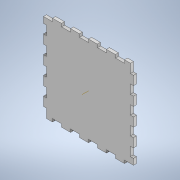
# Autodesk Inventor part: Lukt_hlidarplata
Saved by Autodesk Inventor 2021 (Build 250183000, 183)
## iProperties
Created: 2023-02-22
Part Number: Lukt_hlidarplata
Material: Generic
Document SubType Name: Modeling
Designer: frost
Density: 1 g/cm^3
Appearance: Default
width: 120.000 mm
height: 120.000 mm
thickness: 4.000 mm
finger: 12.000 mm
kerf: 0.220 mm
nr_width: 10.000 ul
nr_height: 10.000 ul
Author: frost
Autodesk Inventor part; units mm, degrees
ref_plane "YZ Plane" through (0, 0, 0) normal (1, 0, 0) x (0, 1, 0)
ref_plane "XZ Plane" through (0, 0, 0) normal (0, 1, 0) x (-1, 0, 0)
ref_plane "XY Plane" through (0, 0, 0) normal (0, 0, 1) x (1, 0, 0)
sketch "Sketch1" plane through (0, 0, 0) normal (0, 0, 1) x (1, 0, 0)
  line L0 (-60, -60) -> (60, -60)
  line L1 (60, -60) -> (60, 60)
  line L2 (60, 60) -> (-60, 60)
  line L3 (-60, 60) -> (-60, -60)
  line L4 (-30, 60) -> (-24.8931, 60)
  point P0 (0, 0)
  dimension "d0" = 120
  dimension "d1" = 120
  dimension "d2" = 60
  dimension "d3" = 60
  constraints: 10 end point, 2 horizontal, 2 parallel, 1 perpendicular, 1 point on line
  measures "d0" distance of L1.end L2.end
  measures "d1" distance of L0.end L1.end
  measures "d2" distance from line of L3 point (0, 0)
  measures "d3" distance from line of L2 point (0, 0)
extrude "Extrusion1" add sketch "Sketch1" along normal mid plane 4
sketch "Sketch3" plane through (-60, 60, 2) normal (0, 1, 0) x (1, 0, 0)
  line L0 (120, 0) -> (0, 0) projected
  line L1 (0, 4) -> (120, 4) projected
  line L2 (0, 0) -> (12, 0)
  line L3 (12, 0) -> (12, 4)
  line L4 (12, 4) -> (0, 4)
  line L5 (0, 4) -> (0, 0)
  line L6 (0, 4) -> (0, 0) projected
  point P0 (60, 2)
  dimension "d17" = 0
  dimension "d18" = 12
  constraints: 8 end point, 2 parallel, 2 point on line, 1 horizontal, 1 perpendicular
  measures "d17" distance between parallel lines of L6 L5
  measures "d18" distance between parallel lines of L3 L5
extrude "Extrusion2" cut sketch "Sketch3" against normal blind 4
pattern_linear "side_top" count 5 spacing 24 along (1, 0, 0) of "Extrusion2"
sketch "Sketch4" plane through (-60, 56, -2) normal (-1, 0, 0) x (0, 0, 1)
  line L0 (4, 0) -> (4, -116) projected
  line L1 (0, -116) -> (4, -116)
  line L2 (4, -116) -> (4, -104)
  line L3 (4, -104) -> (0, -104)
  line L4 (0, -104) -> (0, -116)
  line L5 (0, -116) -> (4, -116) projected
  point P0 (2, -56)
  point P1 (4, -112)
  point P2 (4, -104)
  dimension "d49" = 4
  dimension "d50" = 12
  dimension "d51" = 0
  dimension "d52" = 0
  constraints: 8 end point, 2 parallel, 1 horizontal, 1 perpendicular
  measures "d49" distance of L2.end L3.end
  measures "d50" distance of L3.end L1.start
  measures "d51" distance between parallel lines of L0 L2
  measures "d52" distance between parallel lines of L5 L1
extrude "Extrusion3" cut sketch "Sketch4" against normal blind 4
pattern_circular "side_bottom" count 2 over 360 about axis through (0, 0, -10) along (0, 0, 1) of "Extrusion2", "side_top"
pattern_linear "side_left" count 5 spacing 24 along (0, 1, 0) of "Extrusion3"
pattern_circular "side_right" count 2 over 360 about axis through (0, 0, -10) along (0, 0, 1) of "Extrusion3", "side_left"
sketch "Sketch6" plane through (0, 0, 2) normal (0, 0, 1) x (1, 0, 0)
  line L0 (60, -12) -> (60, 0) projected
  line L1 (60, 0) -> (56, 0) projected
  line L2 (56, 0) -> (56, 12) projected
  line L3 (56, 12) -> (60, 12) projected
  line L4 (60, 12) -> (60, 24) projected
  line L5 (60, 24) -> (56, 24) projected
  line L6 (56, 24) -> (56, 36) projected
  line L7 (56, 36) -> (60, 36) projected
  line L8 (60, 36) -> (60, 48) projected
  line L9 (60, 48) -> (56, 48) projected
  line L10 (56, 48) -> (56, 60) projected
  line L11 (56, 60) -> (48, 60) projected
  line L12 (48, 60) -> (48, 56) projected
  line L13 (48, 56) -> (36, 56) projected
  line L14 (36, 56) -> (36, 60) projected
  line L15 (36, 60) -> (24, 60) projected
  line L16 (24, 60) -> (24, 56) projected
  line L17 (24, 56) -> (12, 56) projected
  line L18 (12, 56) -> (12, 60) projected
  line L19 (12, 60) -> (0, 60) projected
  line L20 (0, 60) -> (0, 56) projected
  line L21 (0, 56) -> (-12, 56) projected
  line L22 (-12, 56) -> (-12, 60) projected
  line L23 (-12, 60) -> (-24, 60) projected
  line L24 (-24, 60) -> (-24, 56) projected
  line L25 (-24, 56) -> (-36, 56) projected
  line L26 (-36, 56) -> (-36, 60) projected
  line L27 (-36, 60) -> (-48, 60) projected
  line L28 (-48, 60) -> (-48, 56) projected
  line L29 (-48, 56) -> (-60, 56) projected
  line L30 (-60, 12) -> (-60, 0) projected
  line L31 (-60, 0) -> (-56, 0) projected
  line L32 (-56, 0) -> (-56, -12) projected
  line L33 (-56, -12) -> (-60, -12) projected
  line L34 (-60, -12) -> (-60, -24) projected
  line L35 (-60, -24) -> (-56, -24) projected
  line L36 (-56, -24) -> (-56, -36) projected
  line L37 (-56, -36) -> (-60, -36) projected
  line L38 (-60, -36) -> (-60, -48) projected
  line L39 (-60, -48) -> (-56, -48) projected
  line L40 (-56, -48) -> (-56, -60) projected
  line L41 (-56, -60) -> (-48, -60) projected
  line L42 (-48, -60) -> (-48, -56) projected
  line L43 (-48, -56) -> (-36, -56) projected
  line L44 (-36, -56) -> (-36, -60) projected
  line L45 (-36, -60) -> (-24, -60) projected
  line L46 (-24, -60) -> (-24, -56) projected
  line L47 (-24, -56) -> (-12, -56) projected
  line L48 (-12, -56) -> (-12, -60) projected
  line L49 (-12, -60) -> (0, -60) projected
  line L50 (0, -60) -> (0, -56) projected
  line L51 (0, -56) -> (12, -56) projected
  line L52 (12, -56) -> (12, -60) projected
  line L53 (12, -60) -> (24, -60) projected
  line L54 (24, -60) -> (24, -56) projected
  line L55 (24, -56) -> (36, -56) projected
  line L56 (36, -56) -> (36, -60) projected
  line L57 (36, -60) -> (48, -60) projected
  line L58 (48, -60) -> (48, -56) projected
  line L59 (48, -56) -> (60, -56) projected
  line L60 (-60.11, 60.11) -> (-35.89, 60.11)
  line L61 (-35.89, 60.11) -> (-35.89, 56.11)
  line L62 (-35.89, 56.11) -> (-24.11, 56.11)
  line L63 (-24.11, 56.11) -> (-24.11, 60.11)
  line L64 (-24.11, 60.11) -> (-11.89, 60.11)
  line L65 (-11.89, 60.11) -> (-11.89, 56.11)
  line L66 (-11.89, 56.11) -> (-0.11, 56.11)
  line L67 (-0.11, 56.11) -> (-0.11, 60.11)
  line L68 (-0.11, 60.11) -> (12.11, 60.11)
  line L69 (12.11, 60.11) -> (12.11, 56.11)
  line L70 (12.11, 56.11) -> (23.89, 56.11)
  line L71 (23.89, 56.11) -> (23.89, 60.11)
  line L72 (23.89, 60.11) -> (36.11, 60.11)
  line L73 (36.11, 60.11) -> (36.11, 56.11)
  line L74 (36.11, 56.11) -> (47.89, 56.11)
  line L75 (47.89, 56.11) -> (47.89, 60.11)
  line L76 (47.89, 60.11) -> (56.11, 60.11)
  line L77 (56.11, 60.11) -> (56.11, 48.11)
  line L78 (56.11, 48.11) -> (60.11, 48.11)
  line L79 (60.11, 48.11) -> (60.11, 35.89)
  line L80 (60.11, 35.89) -> (56.11, 35.89)
  line L81 (56.11, 35.89) -> (56.11, 24.11)
  line L82 (56.11, 24.11) -> (60.11, 24.11)
  line L83 (60.11, 24.11) -> (60.11, 11.89)
  line L84 (60.11, 11.89) -> (56.11, 11.89)
  line L85 (56.11, 11.89) -> (56.11, 0.11)
  line L86 (56.11, 0.11) -> (60.11, 0.11)
  line L87 (60.11, 0.11) -> (60.11, -22.11)
  line L88 (60.11, -22.11) -> (56.11, -22.11)
  line L89 (56.11, -22.11) -> (56.11, -33.89)
  line L90 (56.11, -33.89) -> (60.11, -33.89)
  line L91 (60.11, -33.89) -> (60.11, -24.11)
  line L92 (60.11, -24.11) -> (56.11, -24.11)
  line L93 (56.11, -24.11) -> (56.11, -35.89)
  line L94 (56.11, -35.89) -> (60.11, -35.89)
  line L95 (60.11, -35.89) -> (60.11, -68.11)
  line L96 (60.11, -68.11) -> (60.11, -68.11)
  line L97 (60.11, -68.11) -> (60.11, -72.11)
  line L98 (60.11, -72.11) -> (23.89, -72.11)
  line L99 (23.89, -72.11) -> (23.89, -68.11)
  line L100 (23.89, -68.11) -> (36.11, -68.11)
  line L101 (36.11, -68.11) -> (36.11, -72.11)
  line L102 (36.11, -72.11) -> (-0.11, -72.11)
  line L103 (-0.11, -72.11) -> (-0.11, -68.11)
  line L104 (-0.11, -68.11) -> (12.11, -68.11)
  line L105 (12.11, -68.11) -> (12.11, -72.11)
  line L106 (12.11, -72.11) -> (-24.11, -72.11)
  line L107 (-24.11, -72.11) -> (-24.11, -68.11)
  line L108 (-24.11, -68.11) -> (-11.89, -68.11)
  line L109 (-11.89, -68.11) -> (-11.89, -72.11)
  line L110 (-11.89, -72.11) -> (-48.11, -72.11)
  line L111 (-48.11, -72.11) -> (-48.11, -68.11)
  line L112 (-48.11, -68.11) -> (-35.89, -68.11)
  line L113 (-35.89, -68.11) -> (-35.89, -72.11)
  line L114 (-35.89, -72.11) -> (-68.11, -72.11)
  line L115 (-68.11, -72.11) -> (-68.11, -60.11)
  line L116 (-68.11, -60.11) -> (-72.11, -60.11)
  line L117 (-72.11, -60.11) -> (-72.11, -23.89)
  line L118 (-72.11, -23.89) -> (-68.11, -23.89)
  line L119 (-68.11, -23.89) -> (-68.11, -36.11)
  line L120 (-68.11, -36.11) -> (-72.11, -36.11)
  line L121 (-72.11, -36.11) -> (-72.11, 0.11)
  line L122 (-72.11, 0.11) -> (-68.11, 0.11)
  line L123 (-68.11, 0.11) -> (-68.11, -12.11)
  line L124 (-68.11, -12.11) -> (-72.11, -12.11)
  line L125 (-72.11, -12.11) -> (-72.11, 44.11)
  line L126 (-72.11, 44.11) -> (-68.11, 44.11)
  line L127 (-68.11, 44.11) -> (-68.11, 11.89)
  line L128 (-68.11, 11.89) -> (-72.11, 11.89)
  line L129 (-72.11, 11.89) -> (-72.11, 24.11)
  line L130 (-72.11, 24.11) -> (-68.11, 24.11)
  line L131 (-68.11, 24.11) -> (-68.11, 35.89)
  line L132 (-68.11, 35.89) -> (-72.11, 35.89)
  line L133 (-72.11, 35.89) -> (-72.11, 68.11)
  line L134 (-72.11, 68.11) -> (-60.11, 68.11)
  line L135 (-60.11, 68.11) -> (-60.11, 60.11)
  line L136 (56, -36) -> (60, -36) projected
  line L137 (60, -36) -> (60, -24) projected
  line L138 (60, -24) -> (56, -24) projected
  line L139 (56, -24) -> (56, -12) projected
  line L140 (56, -12) -> (60, -12) projected
  line L141 (-60, 56) -> (-60, 48) projected
  line L142 (-60, 48) -> (-56, 48) projected
  line L143 (-56, 48) -> (-56, 36) projected
  line L144 (-56, 36) -> (-60, 36) projected
  line L145 (-60, 36) -> (-60, 24) projected
  line L146 (-60, 24) -> (-56, 24) projected
  line L147 (-56, 24) -> (-56, 12) projected
  line L148 (-56, 12) -> (-60, 12) projected
  line L149 (60, -56) -> (60, -48) projected
  line L150 (60, -48) -> (56, -48) projected
  line L151 (56, -48) -> (56, -36) projected
  point P0 (0, 0)
  dimension "d59" = 0.11
  constraints: 152 end point, 57 other
  measures "d59" distance between parallel lines of L27 L60
extrude "Extrusion5" [suppressed]
sketch "Sketch7" plane through (0, 0, 2) normal (0, 0, 1) x (1, 0, 0)
  line L0 (-60.11, 68.11) -> (-72.11, 68.11) projected
  line L1 (-72.11, 68.11) -> (-72.11, 35.89) projected
  line L2 (-72.11, 35.89) -> (-68.11, 35.89) projected
  line L3 (-68.11, 35.89) -> (-68.11, 24.11) projected
  line L4 (-68.11, 24.11) -> (-72.11, 24.11) projected
  line L5 (-72.11, 24.11) -> (-72.11, 11.89) projected
  line L6 (-72.11, 11.89) -> (-68.11, 11.89) projected
  line L7 (-68.11, 11.89) -> (-68.11, 0.11) projected
  line L8 (-68.11, 0.11) -> (-72.11, 0.11) projected
  line L9 (-72.11, 0.11) -> (-72.11, -12.11) projected
  line L10 (-72.11, -12.11) -> (-68.11, -12.11) projected
  line L11 (-68.11, -12.11) -> (-68.11, -23.89) projected
  line L12 (-68.11, -23.89) -> (-72.11, -23.89) projected
  line L13 (-72.11, -23.89) -> (-72.11, -36.11) projected
  line L14 (-72.11, -36.11) -> (-68.11, -36.11) projected
  line L15 (-68.11, -36.11) -> (-68.11, -47.89) projected
  line L16 (-68.11, -47.89) -> (-72.11, -47.89) projected
  line L17 (-72.11, -47.89) -> (-72.11, -60.11) projected
  line L18 (-72.11, -60.11) -> (-68.11, -60.11) projected
  line L19 (-68.11, -60.11) -> (-68.11, -72.11) projected
  line L20 (-68.11, -72.11) -> (-35.89, -72.11) projected
  line L21 (-35.89, -72.11) -> (-35.89, -68.11) projected
  line L22 (-35.89, -68.11) -> (-24.11, -68.11) projected
  line L23 (-24.11, -68.11) -> (-24.11, -72.11) projected
  line L24 (-24.11, -72.11) -> (-11.89, -72.11) projected
  line L25 (-11.89, -72.11) -> (-11.89, -68.11) projected
  line L26 (-11.89, -68.11) -> (-0.11, -68.11) projected
  line L27 (-0.11, -68.11) -> (-0.11, -72.11) projected
  line L28 (-0.11, -72.11) -> (12.11, -72.11) projected
  line L29 (12.11, -72.11) -> (12.11, -68.11) projected
  line L30 (12.11, -68.11) -> (23.89, -68.11) projected
  line L31 (23.89, -68.11) -> (23.89, -72.11) projected
  line L32 (23.89, -72.11) -> (36.11, -72.11) projected
  line L33 (36.11, -72.11) -> (36.11, -68.11) projected
  line L34 (36.11, -68.11) -> (47.89, -68.11) projected
  line L35 (47.89, -68.11) -> (47.89, -72.11) projected
  line L36 (47.89, -72.11) -> (60.11, -72.11) projected
  line L37 (60.11, -72.11) -> (60.11, -68.11) projected
  line L38 (60.11, -68.11) -> (72.11, -68.11) projected
  line L39 (72.11, -68.11) -> (72.11, -35.89) projected
  line L40 (72.11, -35.89) -> (68.11, -35.89) projected
  line L41 (68.11, -35.89) -> (68.11, -24.11) projected
  line L42 (68.11, -24.11) -> (72.11, -24.11) projected
  line L43 (72.11, -24.11) -> (72.11, -11.89) projected
  line L44 (72.11, -11.89) -> (68.11, -11.89) projected
  line L45 (68.11, -11.89) -> (68.11, -0.11) projected
  line L46 (68.11, -0.11) -> (72.11, -0.11) projected
  line L47 (72.11, -0.11) -> (72.11, 12.11) projected
  line L48 (72.11, 12.11) -> (68.11, 12.11) projected
  line L49 (68.11, 12.11) -> (68.11, 23.89) projected
  line L50 (68.11, 23.89) -> (72.11, 23.89) projected
  line L51 (72.11, 23.89) -> (72.11, 36.11) projected
  line L52 (72.11, 36.11) -> (68.11, 36.11) projected
  line L53 (68.11, 36.11) -> (68.11, 47.89) projected
  line L54 (68.11, 47.89) -> (72.11, 47.89) projected
  line L55 (72.11, 47.89) -> (72.11, 60.11) projected
  line L56 (72.11, 60.11) -> (68.11, 60.11) projected
  line L57 (68.11, 60.11) -> (68.11, 72.11) projected
  line L58 (68.11, 72.11) -> (35.89, 72.11) projected
  line L59 (35.89, 72.11) -> (35.89, 68.11) projected
  line L60 (35.89, 68.11) -> (24.11, 68.11) projected
  line L61 (24.11, 68.11) -> (24.11, 72.11) projected
  line L62 (24.11, 72.11) -> (11.89, 72.11) projected
  line L63 (11.89, 72.11) -> (11.89, 68.11) projected
  line L64 (11.89, 68.11) -> (0.11, 68.11) projected
  line L65 (0.11, 68.11) -> (0.11, 72.11) projected
  line L66 (0.11, 72.11) -> (-12.11, 72.11) projected
  line L67 (-12.11, 72.11) -> (-12.11, 68.11) projected
  line L68 (-12.11, 68.11) -> (-23.89, 68.11) projected
  line L69 (-23.89, 68.11) -> (-23.89, 72.11) projected
  line L70 (-23.89, 72.11) -> (-36.11, 72.11) projected
  line L71 (-36.11, 72.11) -> (-36.11, 68.11) projected
  line L72 (-36.11, 68.11) -> (-47.89, 68.11) projected
  line L73 (-47.89, 68.11) -> (-47.89, 72.11) projected
  line L74 (-47.89, 72.11) -> (-60.11, 72.11) projected
  line L75 (-60.11, 72.11) -> (-60.11, 68.11) projected
  point P0 (0, 0)
equation "\"d0\" = width"
equation "\"d1\" = height"
equation "\"d2\" = 0.5 * width"
equation "\"d3\" = 0.5 * height"
equation "\"d4\" = thickness"
equation "\"d18\" = finger"
equation "\"d19\" = thickness"
equation "\"d23\" = 2 * finger"
equation "\"d49\" = thickness"
equation "\"d50\" = finger"
equation "\"d28\" = thickness"
equation "\"d55\" = 2 * finger"
equation "\"d59\" = 0.5 * kerf"
equation "\"d60\" = thickness"
equation "\"width\" = 120"
equation "\"height\" = 120"
equation "\"thickness\" = 4"
equation "\"finger\" = 3 * thickness"
equation "\"kerf\" = 0.22"
body "Solid1"
